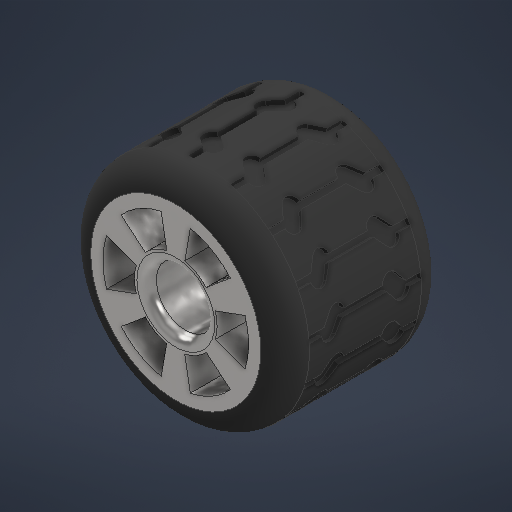
# Autodesk Inventor part: opona
Saved by Autodesk Inventor 2026.2 (Build 302298000, 298)
## iProperties
Created: 2026-08-15
Part Number: opona
Material: Tworzywo sztuczne ABS
Document SubType Name: Modeling
Designer: wojsl
Density: 1.06 g/cm^3
Appearance: Gładki — biały
Author: wojsl
Autodesk Inventor part; units mm, degrees
ref_plane "YZ Plane" through (0, 0, 0) normal (1, 0, 0) x (0, 1, 0)
ref_plane "XZ Plane" through (0, 0, 0) normal (0, 1, 0) x (-1, 0, 0)
sketch "Szkic2" plane through (0, 0, 0) normal (0, 0, 1) x (1, 0, 0)
  circle A0 centre (0, 0) radius 2.25
  dimension "d0" = 4.5
  constraints: 1 centre point, 1 coincident
  measures "d0" diameter of A0
extrude "Wyciągnięcie proste1" add sketch "Szkic2" along normal blind 3.3
fillet "Zaokrąglenie1" radius 0.5 1 edges at (-2.25, 0, 3.3)
fillet "Zaokrąglenie2" radius 0.5 1 edges at (-2.25, 0, 0)
sketch "Szkic3" plane through (0, 0, 0) normal (0, 0, -1) x (-1, 0, 0)
  circle A0 centre (0, 0) radius 0.6
  dimension "d5" = 1.2
  constraints: 1 centre point, 1 coincident
  measures "d5" diameter of A0
extrude "Wyciągnięcie proste2" cut sketch "Szkic3" against normal through all
sketch "Szkic4" plane through (0, 0, 0) normal (0, 0, -1) x (-1, 0, 0)
  circle A0 centre (0, 0) radius 0.75
  circle A1 centre (0, 0) radius 1.75
  dimension "d8" = 1.5
  dimension "d9" = 3.5
  constraints: 2 centre point, 2 coincident
  measures "d8" diameter of A0
  measures "d9" diameter of A1
extrude "Wyciągnięcie proste3" cut sketch "Szkic4" against normal blind 0.5
fillet "Zaokrąglenie3" radius 0.5 1 edges at (0.75, 0, 0)
chamfer "Faza3" distance 1 angle 20 1 edges at (1.75, 0, 0.5) measured on face at (1.25, 0, 0.5)
sketch "Szkic6" plane through (0, 0, 3.3) normal (0, 0, 1) x (1, 0, 0)
  arc A0 (0.8111, -0.2543) -> (0.8111, 0.2543) centre (0, 0) ccw
  arc A1 (1.4222, -0.4767) -> (1.4222, 0.4767) centre (0, 0) ccw
  line L0 (0.85, 0) -> (1.5, 0)
  line L1 (0.8111, 0.2543) -> (1.4222, 0.4767)
  line L2 (0.8111, -0.2543) -> (1.4222, -0.4767)
  dimension "d22" = 1.7
  dimension "d23" = 3
  dimension "d24" = 20
  dimension "d25" = 20
  constraints: 6 end point, 6 point on circle, 2 centre point, 2 coincident, 1 horizontal
  measures "d22" diameter of A0
  measures "d23" diameter of A1
  measures "d24" angle of L0 L1
  measures "d25" angle of L2 L0
extrude "Wyciągnięcie proste4" cut sketch "Szkic6" against normal through all
pattern_circular "Szyk kołowy1" count 6 over 360 about axis through (0, 0, 0.3571) along (0, 0, 1) of "Wyciągnięcie proste4"
ref_plane "Płaszczyzna konstrukcyjna1" through (-2.2158, -0.3907, 0) normal (-0.9848078, -0.1736482, 0) x (0, 0, 1)
sketch "Szkic7" plane through (-2.2158, -0.3907, 0) normal (-0.9848078, -0.1736482, 0) x (0, 0, 1)
  line L0 (1.1009, 0.0054) -> (0.8991, 0.2595) construction
  line L1 (0.978, -0.0922) -> (0.7762, 0.1619)
  line L2 (1.022, 0.3572) -> (1.2238, 0.103)
  arc A0 (0.978, -0.0922) -> (1.2238, 0.103) centre (1.1009, 0.0054) ccw
  arc A1 (1.022, 0.3572) -> (0.7762, 0.1619) centre (0.8991, 0.2595) ccw
  line L3 (2.2081, 0.0054) -> (2.3919, 0.2595) construction
  line L4 (2.331, -0.0836) -> (2.5149, 0.1706)
  line L5 (2.269, 0.3485) -> (2.0851, 0.0943)
  arc A2 (2.0851, 0.0943) -> (2.331, -0.0836) centre (2.2081, 0.0054) ccw
  arc A3 (2.5149, 0.1706) -> (2.269, 0.3485) centre (2.3919, 0.2595) ccw
  line L6 (0.5, 2.25) -> (0.5, -2.25) projected
  line L7 (2.8, -2.25) -> (2.8, 2.25) projected
  line L8 (1, 0.1325) -> (0.5, 0.1325)
  line L9 (0.8991, 0.2595) -> (0.5, 0.2595)
  line L10 (2.3, 0.1325) -> (2.8, 0.1325)
  line L11 (2.3919, 0.2595) -> (2.8, 0.2595)
  line L12 (1.1009, 0.0054) -> (2.2081, 0.0054)
  line L13 (2.3, 0.1325) -> (1, 0.1325)
  point P0 (0, 0)
  point P1 (0.8015, 0.3825)
  point P2 (1.1985, -0.1175)
  point P3 (2.1191, -0.1175)
  point P4 (2.4809, 0.3825)
  point P5 (2.5437, 0.2595)
  point P6 (2.4873, 0.1325)
  point P7 (0.7421, 0.2595)
  point P8 (0.7995, 0.1325)
  point P9 (2.1127, 0.1325)
  point P10 (1.2005, 0.1325)
  point P11 (1.2579, 0.0054)
  point P12 (2.0563, 0.0054)
  dimension "d31" = -0.5
  dimension "d32" = 0.5
  dimension "d33" = 0.5
  dimension "d34" = 0.5
  constraints: 28 end point, 12 point on circle, 8 tangent, 5 point on line, 4 centre point, 3 parallel, 3 perpendicular, 2 midpoint, 1 horizontal
  measures "d31" distance from line of L6 L8.start
  measures "d32" distance from line of L7 L10.start
  measures "d33" vertical distance of point (0.801, 0.382) point (1.199, -0.118)
  measures "d34" vertical distance of point (2.119, -0.118) point (2.481, 0.382)
extrude "Wyciągnięcie proste5" cut sketch "Szkic7" against normal blind 0.1
pattern_circular "Szyk kołowy2" count 16 over 360 about axis through (0, 0, 0) along (0, 0, 1) of "Wyciągnięcie proste5"
fillet "Zaokrąglenie4" radius 0.2 1 edges at (1.75, 0, 0.1361)
fillet "Zaokrąglenie5" radius 0.2 1 edges at (0.6, 0, 3.3)
